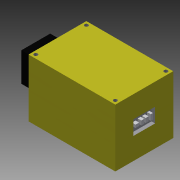
# Autodesk Inventor part: prismatic
Saved by Autodesk Inventor 2015 (Build 190159000, 159)
## iProperties
Created: 2014-11-09
Part Number: prismatic
Material: Generic
Document SubType Name: Modeling
Designer: ericd_000
Density: 1 g/cm^3
Appearance: Default
Author: ericd_000
Autodesk Inventor part; units mm, degrees
ref_plane "YZ Plane" through (0, 0, 0) normal (1, 0, 0) x (0, 1, 0)
ref_plane "XZ Plane" through (0, 0, 0) normal (0, 1, 0) x (-1, 0, 0)
ref_plane "XY Plane" through (0, 0, 0) normal (0, 0, 1) x (1, 0, 0)
sketch "Sketch1" plane through (0, 0, 0) normal (0, 0, 1) x (1, 0, 0)
  line L0 (-60, 40) -> (60, 40)
  line L1 (60, 40) -> (60, -40)
  line L2 (60, -40) -> (-60, -40)
  line L3 (-60, -40) -> (-60, 40)
  point P0 (0, 0)
  point P1 (0, 40)
  point P2 (-60, 0)
  dimension "d0" = 120
  dimension "d1" = 80
  constraints: 8 end point, 2 midpoint, 2 parallel, 1 horizontal, 1 horizontal alignment, 1 perpendicular, 1 vertical alignment
  measures "d0" distance of L0.start L0.end
  measures "d1" distance of L2.end L0.start
extrude "Extrusion1" add sketch "Sketch1" along normal blind 80
sketch "Sketch2" plane through (-60, -40, 0) normal (-1, 0, 0) x (0, 0, 1)
  line L0 (60, 60) -> (20, 60)
  line L1 (20, 60) -> (20, 20)
  line L2 (20, 20) -> (60, 20)
  line L3 (60, 20) -> (60, 60)
  line L4 (0, 0) -> (0, 80) projected
  line L5 (0, 80) -> (80, 80) projected
  point P0 (0, 40)
  point P1 (60, 40)
  point P2 (0, 40)
  point P3 (40, 60)
  point P4 (40, 80)
  dimension "d4" = 40
  dimension "d5" = 40
  constraints: 8 end point, 4 midpoint, 2 parallel, 1 horizontal, 1 horizontal alignment, 1 perpendicular, 1 vertical alignment
  measures "d4" distance of L2.end L0.start
  measures "d5" distance of L0.start L0.end
extrude "Extrusion2" add sketch "Sketch2" along normal blind 30
sketch "Sketch3" plane through (60, -40, 0) normal (1, 0, 0) x (0, 0, -1)
  line L0 (-50, 25) -> (-30, 25)
  line L1 (-30, 25) -> (-30, 55)
  line L2 (-30, 55) -> (-50, 55)
  line L3 (-50, 55) -> (-50, 25)
  line L4 (0, 0) -> (-80, 0)
  line L5 (-80, 0) -> (-80, 80)
  line L6 (-38, 33) -> (-42, 33)
  line L7 (-42, 33) -> (-42, 28)
  line L8 (-42, 28) -> (-38, 28)
  line L9 (-38, 28) -> (-38, 33)
  line L10 (-37, 40) -> (-43, 40)
  line L11 (-43, 40) -> (-43, 36)
  line L12 (-43, 36) -> (-37, 36)
  line L13 (-37, 36) -> (-37, 40)
  line L14 (-37, 46) -> (-43, 46)
  line L15 (-43, 46) -> (-43, 42)
  line L16 (-43, 42) -> (-37, 42)
  line L17 (-37, 42) -> (-37, 46)
  line L18 (-44, 49) -> (-36, 49)
  line L19 (-36, 49) -> (-36, 52)
  line L20 (-36, 52) -> (-44, 52)
  line L21 (-44, 52) -> (-44, 49)
  point P0 (0, 40)
  point P1 (-40, 25)
  point P2 (-40, 0)
  point P3 (-50, 40)
  point P4 (-80, 40)
  point P5 (-40, 28)
  point P6 (-40, 36)
  point P7 (-40, 42)
  point P8 (-40, 52)
  point P9 (-40, 55)
  dimension "d21" = 30
  dimension "d20" = 20
  dimension "d19" = 5
  dimension "d18" = 4
  dimension "d16" = 4
  dimension "d15" = 6
  dimension "d13" = 6
  dimension "d12" = 4
  dimension "d9" = 3
  dimension "d10" = 8
  dimension "d14" = 3
  dimension "d11" = 2
  dimension "d8" = 3
  dimension "d17" = 3
  constraints: 44 end point, 10 parallel, 9 midpoint, 5 horizontal, 5 perpendicular, 5 vertical alignment, 1 horizontal alignment
  measures "d21" distance of L2.end L0.start
  measures "d20" distance of L1.end L2.end
  measures "d19" distance of L6.end L7.end
  measures "d18" distance of L7.end L8.end
  measures "d16" distance of L10.end L11.end
  measures "d15" distance of L10.start L10.end
  measures "d13" distance of L14.start L14.end
  measures "d12" distance of L14.end L15.end
  measures "d9" distance of L20.end L18.start
  measures "d10" distance of L18.start L18.end
  measures "d14" distance between parallel lines of L12 L6
  measures "d11" distance between parallel lines of L16 L10
  measures "d8" distance between parallel lines of L18 L14
  measures "d17" distance between parallel lines of L0 L8
extrude "Extrusion3" cut sketch "Sketch3" against normal blind 5
sketch "Sketch4" plane through (0, 0, 80) normal (0, 0, 1) x (1, 0, 0)
  circle A0 centre (55, 35) radius 2.5
  line L0 (60, 40) -> (-60, 40) projected
  line L1 (60, -40) -> (60, 40) projected
  circle A1 centre (55, -35) radius 2.5
  circle A2 centre (-55, 35) radius 2.5
  circle A3 centre (-55, -35) radius 2.5
  point P0 (0, 0)
  dimension "d25" = 5
  dimension "d26" = 5
  dimension "d27" = 5
  dimension "d30" = 70
  dimension "d33" = 110
  constraints: 4 centre point, 1 horizontal, 1 vertical, 6 other
  measures "d25" diameter of A0
  measures "d26" distance from line of L0 A0.centre
  measures "d27" distance from line of L1 A0.centre
  measures "d30" distance of A0.centre A1.centre
  measures "d33" distance of A0.centre A2.centre
extrude "Extrusion4" cut sketch "Sketch4" against normal blind 5
body "Solid1"
